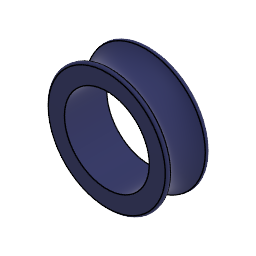
BearingSleeve_v5 (Autodesk Fusion 360 design; units mm, degrees)
Autodesk Fusion 360 part; units mm, degrees
sketch "Sketch1" plane through (0, 0, 0) normal (0, 0, 1) x (1, 0, 0)
  line L0 (0, 0) -> (-4.1, 0) construction
  line L1 (-4.1, 2) -> (-4.1, -2)
  line L2 (-4.1, 2) -> (-6.5, 2)
  line L3 (-6.5, 2) -> (-6.5, -2.015)
  line L4 (-6.5, -2.015) -> (-4.1, -2)
  arc A0 (-6.5, -2.015) -> (-6.5, 2) centre (-6.853, -0.0075) ccw
  dimension "d1" = 4.1
  dimension "d2" = 4
  dimension "d3" = 2.4
  constraint coincident L0.start origin
  constraint horizontal L0
  constraint midpoint L0.end L1
  constraint perpendicular L0 L1
  constraint perpendicular L1 L2
  constraint perpendicular L2 L3
  measures "d1" distance of L0.start L0.end
  measures "d2" distance of L1.start L1.end
  measures "d3" distance of L1.start L2.end
revolve "Revolve1" add sketch "Sketch1" angle 360 about axis through (0, 1.75, 0) along (0, 1, 0) contours L1 L2 L4 A0
fillet "Fillet1" radius 0.2 2 edges at (-6.0601, 2, 2.3505) (-6.0601, -2.015, 2.3505)
move_face "OffsetFaces1" offset 0.1 1 faces at (-4.0949, 0.6667, -0.2044)
